Autodesk Inventor part; units mm, degrees
(part 2 of 2)
  line L790 (66.3671, -24) -> (65.1836, -26.05)
  line L791 (65.1836, -26.05) -> (62.8164, -26.05)
  line L792 (62.8164, -26.05) -> (61.6329, -24)
  line L793 (61.6329, -24) -> (62.8164, -21.95)
  circle A263 centre (64, -24) radius 1.1
  circle A264 centre (64, -32) radius 2.05
  line L794 (62.8164, -29.95) -> (65.1836, -29.95)
  line L795 (65.1836, -29.95) -> (66.3671, -32)
  line L796 (66.3671, -32) -> (65.1836, -34.05)
  line L797 (65.1836, -34.05) -> (62.8164, -34.05)
  line L798 (62.8164, -34.05) -> (61.6329, -32)
  line L799 (61.6329, -32) -> (62.8164, -29.95)
  circle A265 centre (64, -32) radius 1.1
  circle A266 centre (64, -40) radius 2.05
  line L800 (62.8164, -37.95) -> (65.1836, -37.95)
  line L801 (65.1836, -37.95) -> (66.3671, -40)
  line L802 (66.3671, -40) -> (65.1836, -42.05)
  line L803 (65.1836, -42.05) -> (62.8164, -42.05)
  line L804 (62.8164, -42.05) -> (61.6329, -40)
  line L805 (61.6329, -40) -> (62.8164, -37.95)
  circle A267 centre (64, -40) radius 1.1
  circle A268 centre (64, -48) radius 2.05
  line L806 (62.8164, -45.95) -> (65.1836, -45.95)
  line L807 (65.1836, -45.95) -> (66.3671, -48)
  line L808 (66.3671, -48) -> (65.1836, -50.05)
  line L809 (65.1836, -50.05) -> (62.8164, -50.05)
  line L810 (62.8164, -50.05) -> (61.6329, -48)
  line L811 (61.6329, -48) -> (62.8164, -45.95)
  circle A269 centre (64, -48) radius 1.1
  circle A270 centre (64, -56) radius 2.05
  line L812 (62.8164, -53.95) -> (65.1836, -53.95)
  line L813 (65.1836, -53.95) -> (66.3671, -56)
  line L814 (66.3671, -56) -> (65.1836, -58.05)
  line L815 (65.1836, -58.05) -> (62.8164, -58.05)
  line L816 (62.8164, -58.05) -> (61.6329, -56)
  line L817 (61.6329, -56) -> (62.8164, -53.95)
  circle A271 centre (64, -56) radius 1.1
  circle A272 centre (64, -64) radius 2.05
  line L818 (62.8164, -61.95) -> (65.1836, -61.95)
  line L819 (65.1836, -61.95) -> (66.3671, -64)
  line L820 (66.3671, -64) -> (65.1836, -66.05)
  line L821 (65.1836, -66.05) -> (62.8164, -66.05)
  line L822 (62.8164, -66.05) -> (61.6329, -64)
  line L823 (61.6329, -64) -> (62.8164, -61.95)
  circle A273 centre (64, -64) radius 1.1
  circle A274 centre (64, -72) radius 2.05
  line L824 (62.8164, -69.95) -> (65.1836, -69.95)
  line L825 (65.1836, -69.95) -> (66.3671, -72)
  line L826 (66.3671, -72) -> (65.1836, -74.05)
  line L827 (65.1836, -74.05) -> (62.8164, -74.05)
  line L828 (62.8164, -74.05) -> (61.6329, -72)
  line L829 (61.6329, -72) -> (62.8164, -69.95)
  circle A275 centre (64, -72) radius 1.1
  circle A276 centre (64, -80) radius 2.05
  line L830 (62.8164, -77.95) -> (65.1836, -77.95)
  line L831 (65.1836, -77.95) -> (66.3671, -80)
  line L832 (66.3671, -80) -> (65.1836, -82.05)
  line L833 (65.1836, -82.05) -> (62.8164, -82.05)
  line L834 (62.8164, -82.05) -> (61.6329, -80)
  line L835 (61.6329, -80) -> (62.8164, -77.95)
  circle A277 centre (64, -80) radius 1.1
  circle A278 centre (64, -88) radius 2.05
  line L836 (62.8164, -85.95) -> (65.1836, -85.95)
  line L837 (65.1836, -85.95) -> (66.3671, -88)
  line L838 (66.3671, -88) -> (65.1836, -90.05)
  line L839 (65.1836, -90.05) -> (62.8164, -90.05)
  line L840 (62.8164, -90.05) -> (61.6329, -88)
  line L841 (61.6329, -88) -> (62.8164, -85.95)
  circle A279 centre (64, -88) radius 1.1
  circle A280 centre (64, -96) radius 2.05
  line L842 (62.8164, -93.95) -> (65.1836, -93.95)
  line L843 (65.1836, -93.95) -> (66.3671, -96)
  line L844 (66.3671, -96) -> (65.1836, -98.05)
  line L845 (65.1836, -98.05) -> (62.8164, -98.05)
  line L846 (62.8164, -98.05) -> (61.6329, -96)
  line L847 (61.6329, -96) -> (62.8164, -93.95)
  circle A281 centre (64, -96) radius 1.1
  circle A282 centre (64, -104) radius 2.05
  line L848 (62.8164, -101.95) -> (65.1836, -101.95)
  line L849 (65.1836, -101.95) -> (66.3671, -104)
  line L850 (66.3671, -104) -> (65.1836, -106.05)
  line L851 (65.1836, -106.05) -> (62.8164, -106.05)
  line L852 (62.8164, -106.05) -> (61.6329, -104)
  line L853 (61.6329, -104) -> (62.8164, -101.95)
  circle A283 centre (64, -104) radius 1.1
  circle A284 centre (64, -112) radius 2.05
  line L854 (62.8164, -109.95) -> (65.1836, -109.95)
  line L855 (65.1836, -109.95) -> (66.3671, -112)
  line L856 (66.3671, -112) -> (65.1836, -114.05)
  line L857 (65.1836, -114.05) -> (62.8164, -114.05)
  line L858 (62.8164, -114.05) -> (61.6329, -112)
  line L859 (61.6329, -112) -> (62.8164, -109.95)
  circle A285 centre (64, -112) radius 1.1
  circle A286 centre (64, -120) radius 2.05
  line L860 (62.8164, -117.95) -> (65.1836, -117.95)
  line L861 (65.1836, -117.95) -> (66.3671, -120)
  line L862 (66.3671, -120) -> (65.1836, -122.05)
  line L863 (65.1836, -122.05) -> (62.8164, -122.05)
  line L864 (62.8164, -122.05) -> (61.6329, -120)
  line L865 (61.6329, -120) -> (62.8164, -117.95)
  circle A287 centre (64, -120) radius 1.1
  circle A288 centre (72, 0) radius 2.05
  line L866 (70.8164, 2.05) -> (73.1836, 2.05)
  line L867 (73.1836, 2.05) -> (74.3671, 0)
  line L868 (74.3671, 0) -> (73.1836, -2.05)
  line L869 (73.1836, -2.05) -> (70.8164, -2.05)
  line L870 (70.8164, -2.05) -> (69.6329, 0)
  line L871 (69.6329, 0) -> (70.8164, 2.05)
  circle A289 centre (72, 0) radius 1.1
  circle A290 centre (72, -8) radius 2.05
  line L872 (70.8164, -5.95) -> (73.1836, -5.95)
  line L873 (73.1836, -5.95) -> (74.3671, -8)
  line L874 (74.3671, -8) -> (73.1836, -10.05)
  line L875 (73.1836, -10.05) -> (70.8164, -10.05)
  line L876 (70.8164, -10.05) -> (69.6329, -8)
  line L877 (69.6329, -8) -> (70.8164, -5.95)
  circle A291 centre (72, -8) radius 1.1
  circle A292 centre (72, -16) radius 2.05
  line L878 (70.8164, -13.95) -> (73.1836, -13.95)
  line L879 (73.1836, -13.95) -> (74.3671, -16)
  line L880 (74.3671, -16) -> (73.1836, -18.05)
  line L881 (73.1836, -18.05) -> (70.8164, -18.05)
  line L882 (70.8164, -18.05) -> (69.6329, -16)
  line L883 (69.6329, -16) -> (70.8164, -13.95)
  circle A293 centre (72, -16) radius 1.1
  circle A294 centre (72, -24) radius 2.05
  line L884 (70.8164, -21.95) -> (73.1836, -21.95)
  line L885 (73.1836, -21.95) -> (74.3671, -24)
  line L886 (74.3671, -24) -> (73.1836, -26.05)
  line L887 (73.1836, -26.05) -> (70.8164, -26.05)
  line L888 (70.8164, -26.05) -> (69.6329, -24)
  line L889 (69.6329, -24) -> (70.8164, -21.95)
  circle A295 centre (72, -24) radius 1.1
  circle A296 centre (72, -32) radius 2.05
  line L890 (70.8164, -29.95) -> (73.1836, -29.95)
  line L891 (73.1836, -29.95) -> (74.3671, -32)
  line L892 (74.3671, -32) -> (73.1836, -34.05)
  line L893 (73.1836, -34.05) -> (70.8164, -34.05)
  line L894 (70.8164, -34.05) -> (69.6329, -32)
  line L895 (69.6329, -32) -> (70.8164, -29.95)
  circle A297 centre (72, -32) radius 1.1
  circle A298 centre (72, -40) radius 2.05
  line L896 (70.8164, -37.95) -> (73.1836, -37.95)
  line L897 (73.1836, -37.95) -> (74.3671, -40)
  line L898 (74.3671, -40) -> (73.1836, -42.05)
  line L899 (73.1836, -42.05) -> (70.8164, -42.05)
  line L900 (70.8164, -42.05) -> (69.6329, -40)
  line L901 (69.6329, -40) -> (70.8164, -37.95)
  circle A299 centre (72, -40) radius 1.1
  circle A300 centre (72, -48) radius 2.05
  line L902 (70.8164, -45.95) -> (73.1836, -45.95)
  line L903 (73.1836, -45.95) -> (74.3671, -48)
  line L904 (74.3671, -48) -> (73.1836, -50.05)
  line L905 (73.1836, -50.05) -> (70.8164, -50.05)
  line L906 (70.8164, -50.05) -> (69.6329, -48)
  line L907 (69.6329, -48) -> (70.8164, -45.95)
  circle A301 centre (72, -48) radius 1.1
  circle A302 centre (72, -56) radius 2.05
  line L908 (70.8164, -53.95) -> (73.1836, -53.95)
  line L909 (73.1836, -53.95) -> (74.3671, -56)
  line L910 (74.3671, -56) -> (73.1836, -58.05)
  line L911 (73.1836, -58.05) -> (70.8164, -58.05)
  line L912 (70.8164, -58.05) -> (69.6329, -56)
  line L913 (69.6329, -56) -> (70.8164, -53.95)
  circle A303 centre (72, -56) radius 1.1
  circle A304 centre (72, -64) radius 2.05
  line L914 (70.8164, -61.95) -> (73.1836, -61.95)
  line L915 (73.1836, -61.95) -> (74.3671, -64)
  line L916 (74.3671, -64) -> (73.1836, -66.05)
  line L917 (73.1836, -66.05) -> (70.8164, -66.05)
  line L918 (70.8164, -66.05) -> (69.6329, -64)
  line L919 (69.6329, -64) -> (70.8164, -61.95)
  circle A305 centre (72, -64) radius 1.1
  circle A306 centre (72, -72) radius 2.05
  line L920 (70.8164, -69.95) -> (73.1836, -69.95)
  line L921 (73.1836, -69.95) -> (74.3671, -72)
  line L922 (74.3671, -72) -> (73.1836, -74.05)
  line L923 (73.1836, -74.05) -> (70.8164, -74.05)
  line L924 (70.8164, -74.05) -> (69.6329, -72)
  line L925 (69.6329, -72) -> (70.8164, -69.95)
  circle A307 centre (72, -72) radius 1.1
  circle A308 centre (72, -80) radius 2.05
  line L926 (70.8164, -77.95) -> (73.1836, -77.95)
  line L927 (73.1836, -77.95) -> (74.3671, -80)
  line L928 (74.3671, -80) -> (73.1836, -82.05)
  line L929 (73.1836, -82.05) -> (70.8164, -82.05)
  line L930 (70.8164, -82.05) -> (69.6329, -80)
  line L931 (69.6329, -80) -> (70.8164, -77.95)
  circle A309 centre (72, -80) radius 1.1
  circle A310 centre (72, -88) radius 2.05
  line L932 (70.8164, -85.95) -> (73.1836, -85.95)
  line L933 (73.1836, -85.95) -> (74.3671, -88)
  line L934 (74.3671, -88) -> (73.1836, -90.05)
  line L935 (73.1836, -90.05) -> (70.8164, -90.05)
  line L936 (70.8164, -90.05) -> (69.6329, -88)
  line L937 (69.6329, -88) -> (70.8164, -85.95)
  circle A311 centre (72, -88) radius 1.1
  circle A312 centre (72, -96) radius 2.05
  line L938 (70.8164, -93.95) -> (73.1836, -93.95)
  line L939 (73.1836, -93.95) -> (74.3671, -96)
  line L940 (74.3671, -96) -> (73.1836, -98.05)
  line L941 (73.1836, -98.05) -> (70.8164, -98.05)
  line L942 (70.8164, -98.05) -> (69.6329, -96)
  line L943 (69.6329, -96) -> (70.8164, -93.95)
  circle A313 centre (72, -96) radius 1.1
  circle A314 centre (72, -104) radius 2.05
  line L944 (70.8164, -101.95) -> (73.1836, -101.95)
  line L945 (73.1836, -101.95) -> (74.3671, -104)
  line L946 (74.3671, -104) -> (73.1836, -106.05)
  line L947 (73.1836, -106.05) -> (70.8164, -106.05)
  line L948 (70.8164, -106.05) -> (69.6329, -104)
  line L949 (69.6329, -104) -> (70.8164, -101.95)
  circle A315 centre (72, -104) radius 1.1
  circle A316 centre (72, -112) radius 2.05
  line L950 (70.8164, -109.95) -> (73.1836, -109.95)
  line L951 (73.1836, -109.95) -> (74.3671, -112)
  line L952 (74.3671, -112) -> (73.1836, -114.05)
  line L953 (73.1836, -114.05) -> (70.8164, -114.05)
  line L954 (70.8164, -114.05) -> (69.6329, -112)
  line L955 (69.6329, -112) -> (70.8164, -109.95)
  circle A317 centre (72, -112) radius 1.1
  circle A318 centre (72, -120) radius 2.05
  line L956 (70.8164, -117.95) -> (73.1836, -117.95)
  line L957 (73.1836, -117.95) -> (74.3671, -120)
  line L958 (74.3671, -120) -> (73.1836, -122.05)
  line L959 (73.1836, -122.05) -> (70.8164, -122.05)
  line L960 (70.8164, -122.05) -> (69.6329, -120)
  line L961 (69.6329, -120) -> (70.8164, -117.95)
  circle A319 centre (72, -120) radius 1.1
  circle A320 centre (80, 0) radius 2.05
  line L962 (78.8164, 2.05) -> (81.1836, 2.05)
  line L963 (81.1836, 2.05) -> (82.3671, 0)
  line L964 (82.3671, 0) -> (81.1836, -2.05)
  line L965 (81.1836, -2.05) -> (78.8164, -2.05)
  line L966 (78.8164, -2.05) -> (77.6329, 0)
  line L967 (77.6329, 0) -> (78.8164, 2.05)
  circle A321 centre (80, 0) radius 1.1
  circle A322 centre (80, -8) radius 2.05
  line L968 (78.8164, -5.95) -> (81.1836, -5.95)
  line L969 (81.1836, -5.95) -> (82.3671, -8)
  line L970 (82.3671, -8) -> (81.1836, -10.05)
  line L971 (81.1836, -10.05) -> (78.8164, -10.05)
  line L972 (78.8164, -10.05) -> (77.6329, -8)
  line L973 (77.6329, -8) -> (78.8164, -5.95)
  circle A323 centre (80, -8) radius 1.1
  circle A324 centre (80, -16) radius 2.05
  line L974 (78.8164, -13.95) -> (81.1836, -13.95)
  line L975 (81.1836, -13.95) -> (82.3671, -16)
  line L976 (82.3671, -16) -> (81.1836, -18.05)
  line L977 (81.1836, -18.05) -> (78.8164, -18.05)
  line L978 (78.8164, -18.05) -> (77.6329, -16)
  line L979 (77.6329, -16) -> (78.8164, -13.95)
  circle A325 centre (80, -16) radius 1.1
  circle A326 centre (80, -24) radius 2.05
  line L980 (78.8164, -21.95) -> (81.1836, -21.95)
  line L981 (81.1836, -21.95) -> (82.3671, -24)
  line L982 (82.3671, -24) -> (81.1836, -26.05)
  line L983 (81.1836, -26.05) -> (78.8164, -26.05)
  line L984 (78.8164, -26.05) -> (77.6329, -24)
  line L985 (77.6329, -24) -> (78.8164, -21.95)
  circle A327 centre (80, -24) radius 1.1
  circle A328 centre (80, -32) radius 2.05
  line L986 (78.8164, -29.95) -> (81.1836, -29.95)
  line L987 (81.1836, -29.95) -> (82.3671, -32)
  line L988 (82.3671, -32) -> (81.1836, -34.05)
  line L989 (81.1836, -34.05) -> (78.8164, -34.05)
  line L990 (78.8164, -34.05) -> (77.6329, -32)
  line L991 (77.6329, -32) -> (78.8164, -29.95)
  circle A329 centre (80, -32) radius 1.1
  circle A330 centre (80, -40) radius 2.05
  line L992 (78.8164, -37.95) -> (81.1836, -37.95)
  line L993 (81.1836, -37.95) -> (82.3671, -40)
  line L994 (82.3671, -40) -> (81.1836, -42.05)
  line L995 (81.1836, -42.05) -> (78.8164, -42.05)
  line L996 (78.8164, -42.05) -> (77.6329, -40)
  line L997 (77.6329, -40) -> (78.8164, -37.95)
  circle A331 centre (80, -40) radius 1.1
  circle A332 centre (80, -48) radius 2.05
  line L998 (78.8164, -45.95) -> (81.1836, -45.95)
  line L999 (81.1836, -45.95) -> (82.3671, -48)
  line L1000 (82.3671, -48) -> (81.1836, -50.05)
  line L1001 (81.1836, -50.05) -> (78.8164, -50.05)
  line L1002 (78.8164, -50.05) -> (77.6329, -48)
  line L1003 (77.6329, -48) -> (78.8164, -45.95)
  circle A333 centre (80, -48) radius 1.1
  circle A334 centre (80, -56) radius 2.05
  line L1004 (78.8164, -53.95) -> (81.1836, -53.95)
  line L1005 (81.1836, -53.95) -> (82.3671, -56)
  line L1006 (82.3671, -56) -> (81.1836, -58.05)
  line L1007 (81.1836, -58.05) -> (78.8164, -58.05)
  line L1008 (78.8164, -58.05) -> (77.6329, -56)
  line L1009 (77.6329, -56) -> (78.8164, -53.95)
  circle A335 centre (80, -56) radius 1.1
  circle A336 centre (80, -64) radius 2.05
  line L1010 (78.8164, -61.95) -> (81.1836, -61.95)
  line L1011 (81.1836, -61.95) -> (82.3671, -64)
  line L1012 (82.3671, -64) -> (81.1836, -66.05)
  line L1013 (81.1836, -66.05) -> (78.8164, -66.05)
  line L1014 (78.8164, -66.05) -> (77.6329, -64)
  line L1015 (77.6329, -64) -> (78.8164, -61.95)
  circle A337 centre (80, -64) radius 1.1
  circle A338 centre (80, -72) radius 2.05
  line L1016 (78.8164, -69.95) -> (81.1836, -69.95)
  line L1017 (81.1836, -69.95) -> (82.3671, -72)
  line L1018 (82.3671, -72) -> (81.1836, -74.05)
  line L1019 (81.1836, -74.05) -> (78.8164, -74.05)
  line L1020 (78.8164, -74.05) -> (77.6329, -72)
  line L1021 (77.6329, -72) -> (78.8164, -69.95)
  circle A339 centre (80, -72) radius 1.1
  circle A340 centre (80, -80) radius 2.05
  line L1022 (78.8164, -77.95) -> (81.1836, -77.95)
  line L1023 (81.1836, -77.95) -> (82.3671, -80)
  line L1024 (82.3671, -80) -> (81.1836, -82.05)
  line L1025 (81.1836, -82.05) -> (78.8164, -82.05)
  line L1026 (78.8164, -82.05) -> (77.6329, -80)
  line L1027 (77.6329, -80) -> (78.8164, -77.95)
  circle A341 centre (80, -80) radius 1.1
  circle A342 centre (80, -88) radius 2.05
  line L1028 (78.8164, -85.95) -> (81.1836, -85.95)
  line L1029 (81.1836, -85.95) -> (82.3671, -88)
  line L1030 (82.3671, -88) -> (81.1836, -90.05)
  line L1031 (81.1836, -90.05) -> (78.8164, -90.05)
  line L1032 (78.8164, -90.05) -> (77.6329, -88)
  line L1033 (77.6329, -88) -> (78.8164, -85.95)
  circle A343 centre (80, -88) radius 1.1
  circle A344 centre (80, -96) radius 2.05
  line L1034 (78.8164, -93.95) -> (81.1836, -93.95)
  line L1035 (81.1836, -93.95) -> (82.3671, -96)
  line L1036 (82.3671, -96) -> (81.1836, -98.05)
  line L1037 (81.1836, -98.05) -> (78.8164, -98.05)
  line L1038 (78.8164, -98.05) -> (77.6329, -96)
  line L1039 (77.6329, -96) -> (78.8164, -93.95)
  circle A345 centre (80, -96) radius 1.1
  circle A346 centre (80, -104) radius 2.05
  line L1040 (78.8164, -101.95) -> (81.1836, -101.95)
  line L1041 (81.1836, -101.95) -> (82.3671, -104)
  line L1042 (82.3671, -104) -> (81.1836, -106.05)
  line L1043 (81.1836, -106.05) -> (78.8164, -106.05)
  line L1044 (78.8164, -106.05) -> (77.6329, -104)
  line L1045 (77.6329, -104) -> (78.8164, -101.95)
  circle A347 centre (80, -104) radius 1.1
  circle A348 centre (80, -112) radius 2.05
  line L1046 (78.8164, -109.95) -> (81.1836, -109.95)
  line L1047 (81.1836, -109.95) -> (82.3671, -112)
  line L1048 (82.3671, -112) -> (81.1836, -114.05)
  line L1049 (81.1836, -114.05) -> (78.8164, -114.05)
  line L1050 (78.8164, -114.05) -> (77.6329, -112)
  line L1051 (77.6329, -112) -> (78.8164, -109.95)
  circle A349 centre (80, -112) radius 1.1
  circle A350 centre (80, -120) radius 2.05
  line L1052 (78.8164, -117.95) -> (81.1836, -117.95)
  line L1053 (81.1836, -117.95) -> (82.3671, -120)
  line L1054 (82.3671, -120) -> (81.1836, -122.05)
  line L1055 (81.1836, -122.05) -> (78.8164, -122.05)
  line L1056 (78.8164, -122.05) -> (77.6329, -120)
  line L1057 (77.6329, -120) -> (78.8164, -117.95)
  circle A351 centre (80, -120) radius 1.1
  circle A352 centre (88, 0) radius 2.05
  line L1058 (86.8164, 2.05) -> (89.1836, 2.05)
  line L1059 (89.1836, 2.05) -> (90.3671, 0)
  line L1060 (90.3671, 0) -> (89.1836, -2.05)
  line L1061 (89.1836, -2.05) -> (86.8164, -2.05)
  line L1062 (86.8164, -2.05) -> (85.6329, 0)
  line L1063 (85.6329, 0) -> (86.8164, 2.05)
  circle A353 centre (88, 0) radius 1.1
  circle A354 centre (88, -8) radius 2.05
  line L1064 (86.8164, -5.95) -> (89.1836, -5.95)
  line L1065 (89.1836, -5.95) -> (90.3671, -8)
  line L1066 (90.3671, -8) -> (89.1836, -10.05)
  line L1067 (89.1836, -10.05) -> (86.8164, -10.05)
  line L1068 (86.8164, -10.05) -> (85.6329, -8)
  line L1069 (85.6329, -8) -> (86.8164, -5.95)
  circle A355 centre (88, -8) radius 1.1
  circle A356 centre (88, -16) radius 2.05
  line L1070 (86.8164, -13.95) -> (89.1836, -13.95)
  line L1071 (89.1836, -13.95) -> (90.3671, -16)
  line L1072 (90.3671, -16) -> (89.1836, -18.05)
  line L1073 (89.1836, -18.05) -> (86.8164, -18.05)
  line L1074 (86.8164, -18.05) -> (85.6329, -16)
  line L1075 (85.6329, -16) -> (86.8164, -13.95)
  circle A357 centre (88, -16) radius 1.1
  circle A358 centre (88, -24) radius 2.05
  line L1076 (86.8164, -21.95) -> (89.1836, -21.95)
  line L1077 (89.1836, -21.95) -> (90.3671, -24)
  line L1078 (90.3671, -24) -> (89.1836, -26.05)
  line L1079 (89.1836, -26.05) -> (86.8164, -26.05)
  line L1080 (86.8164, -26.05) -> (85.6329, -24)
  line L1081 (85.6329, -24) -> (86.8164, -21.95)
  circle A359 centre (88, -24) radius 1.1
  circle A360 centre (88, -32) radius 2.05
  line L1082 (86.8164, -29.95) -> (89.1836, -29.95)
  line L1083 (89.1836, -29.95) -> (90.3671, -32)
  line L1084 (90.3671, -32) -> (89.1836, -34.05)
  line L1085 (89.1836, -34.05) -> (86.8164, -34.05)
  line L1086 (86.8164, -34.05) -> (85.6329, -32)
  line L1087 (85.6329, -32) -> (86.8164, -29.95)
  circle A361 centre (88, -32) radius 1.1
  circle A362 centre (88, -40) radius 2.05
  line L1088 (86.8164, -37.95) -> (89.1836, -37.95)
  line L1089 (89.1836, -37.95) -> (90.3671, -40)
  line L1090 (90.3671, -40) -> (89.1836, -42.05)
  line L1091 (89.1836, -42.05) -> (86.8164, -42.05)
  line L1092 (86.8164, -42.05) -> (85.6329, -40)
  line L1093 (85.6329, -40) -> (86.8164, -37.95)
  circle A363 centre (88, -40) radius 1.1
  circle A364 centre (88, -48) radius 2.05
  line L1094 (86.8164, -45.95) -> (89.1836, -45.95)
  line L1095 (89.1836, -45.95) -> (90.3671, -48)
  line L1096 (90.3671, -48) -> (89.1836, -50.05)
  line L1097 (89.1836, -50.05) -> (86.8164, -50.05)
  line L1098 (86.8164, -50.05) -> (85.6329, -48)
  line L1099 (85.6329, -48) -> (86.8164, -45.95)
  circle A365 centre (88, -48) radius 1.1
  circle A366 centre (88, -56) radius 2.05
  line L1100 (86.8164, -53.95) -> (89.1836, -53.95)
  line L1101 (89.1836, -53.95) -> (90.3671, -56)
  line L1102 (90.3671, -56) -> (89.1836, -58.05)
  line L1103 (89.1836, -58.05) -> (86.8164, -58.05)
  line L1104 (86.8164, -58.05) -> (85.6329, -56)
  line L1105 (85.6329, -56) -> (86.8164, -53.95)
  circle A367 centre (88, -56) radius 1.1
  circle A368 centre (88, -64) radius 2.05
  line L1106 (86.8164, -61.95) -> (89.1836, -61.95)
  line L1107 (89.1836, -61.95) -> (90.3671, -64)
  line L1108 (90.3671, -64) -> (89.1836, -66.05)
  line L1109 (89.1836, -66.05) -> (86.8164, -66.05)
  line L1110 (86.8164, -66.05) -> (85.6329, -64)
  line L1111 (85.6329, -64) -> (86.8164, -61.95)
  circle A369 centre (88, -64) radius 1.1
  circle A370 centre (88, -72) radius 2.05
  line L1112 (86.8164, -69.95) -> (89.1836, -69.95)
  line L1113 (89.1836, -69.95) -> (90.3671, -72)
  line L1114 (90.3671, -72) -> (89.1836, -74.05)
  line L1115 (89.1836, -74.05) -> (86.8164, -74.05)
  line L1116 (86.8164, -74.05) -> (85.6329, -72)
  line L1117 (85.6329, -72) -> (86.8164, -69.95)
  circle A371 centre (88, -72) radius 1.1
  circle A372 centre (88, -80) radius 2.05
  line L1118 (86.8164, -77.95) -> (89.1836, -77.95)
  line L1119 (89.1836, -77.95) -> (90.3671, -80)
  line L1120 (90.3671, -80) -> (89.1836, -82.05)
  line L1121 (89.1836, -82.05) -> (86.8164, -82.05)
  line L1122 (86.8164, -82.05) -> (85.6329, -80)
  line L1123 (85.6329, -80) -> (86.8164, -77.95)
  circle A373 centre (88, -80) radius 1.1
  circle A374 centre (88, -88) radius 2.05
  line L1124 (86.8164, -85.95) -> (89.1836, -85.95)
  line L1125 (89.1836, -85.95) -> (90.3671, -88)
  line L1126 (90.3671, -88) -> (89.1836, -90.05)
  line L1127 (89.1836, -90.05) -> (86.8164, -90.05)
  line L1128 (86.8164, -90.05) -> (85.6329, -88)
  line L1129 (85.6329, -88) -> (86.8164, -85.95)
  circle A375 centre (88, -88) radius 1.1
  circle A376 centre (88, -96) radius 2.05
  line L1130 (86.8164, -93.95) -> (89.1836, -93.95)
  line L1131 (89.1836, -93.95) -> (90.3671, -96)
  line L1132 (90.3671, -96) -> (89.1836, -98.05)
  line L1133 (89.1836, -98.05) -> (86.8164, -98.05)
  line L1134 (86.8164, -98.05) -> (85.6329, -96)
  line L1135 (85.6329, -96) -> (86.8164, -93.95)
  circle A377 centre (88, -96) radius 1.1
  circle A378 centre (88, -104) radius 2.05
  line L1136 (86.8164, -101.95) -> (89.1836, -101.95)
  line L1137 (89.1836, -101.95) -> (90.3671, -104)
  line L1138 (90.3671, -104) -> (89.1836, -106.05)
  line L1139 (89.1836, -106.05) -> (86.8164, -106.05)
  line L1140 (86.8164, -106.05) -> (85.6329, -104)
  line L1141 (85.6329, -104) -> (86.8164, -101.95)
  circle A379 centre (88, -104) radius 1.1
  circle A380 centre (88, -112) radius 2.05
  line L1142 (86.8164, -109.95) -> (89.1836, -109.95)
  line L1143 (89.1836, -109.95) -> (90.3671, -112)
  line L1144 (90.3671, -112) -> (89.1836, -114.05)
  line L1145 (89.1836, -114.05) -> (86.8164, -114.05)
  line L1146 (86.8164, -114.05) -> (85.6329, -112)
  line L1147 (85.6329, -112) -> (86.8164, -109.95)
  circle A381 centre (88, -112) radius 1.1
  circle A382 centre (88, -120) radius 2.05
  line L1148 (86.8164, -117.95) -> (89.1836, -117.95)
  line L1149 (89.1836, -117.95) -> (90.3671, -120)
  line L1150 (90.3671, -120) -> (89.1836, -122.05)
  line L1151 (89.1836, -122.05) -> (86.8164, -122.05)
  line L1152 (86.8164, -122.05) -> (85.6329, -120)
  line L1153 (85.6329, -120) -> (86.8164, -117.95)
  circle A383 centre (88, -120) radius 1.1
  circle A384 centre (96, 0) radius 2.05
  line L1154 (94.8164, 2.05) -> (97.1836, 2.05)
  line L1155 (97.1836, 2.05) -> (98.3671, 0)
  line L1156 (98.3671, 0) -> (97.1836, -2.05)
  line L1157 (97.1836, -2.05) -> (94.8164, -2.05)
  line L1158 (94.8164, -2.05) -> (93.6329, 0)
  line L1159 (93.6329, 0) -> (94.8164, 2.05)
  circle A385 centre (96, 0) radius 1.1
  circle A386 centre (96, -8) radius 2.05
  line L1160 (94.8164, -5.95) -> (97.1836, -5.95)
  line L1161 (97.1836, -5.95) -> (98.3671, -8)
  line L1162 (98.3671, -8) -> (97.1836, -10.05)
  line L1163 (97.1836, -10.05) -> (94.8164, -10.05)
  line L1164 (94.8164, -10.05) -> (93.6329, -8)
  line L1165 (93.6329, -8) -> (94.8164, -5.95)
  circle A387 centre (96, -8) radius 1.1
  circle A388 centre (96, -16) radius 2.05
  line L1166 (94.8164, -13.95) -> (97.1836, -13.95)
  line L1167 (97.1836, -13.95) -> (98.3671, -16)
  line L1168 (98.3671, -16) -> (97.1836, -18.05)
  line L1169 (97.1836, -18.05) -> (94.8164, -18.05)
  line L1170 (94.8164, -18.05) -> (93.6329, -16)
  line L1171 (93.6329, -16) -> (94.8164, -13.95)
  circle A389 centre (96, -16) radius 1.1
  circle A390 centre (96, -24) radius 2.05
  line L1172 (94.8164, -21.95) -> (97.1836, -21.95)
  line L1173 (97.1836, -21.95) -> (98.3671, -24)
  line L1174 (98.3671, -24) -> (97.1836, -26.05)
  line L1175 (97.1836, -26.05) -> (94.8164, -26.05)
  line L1176 (94.8164, -26.05) -> (93.6329, -24)
  line L1177 (93.6329, -24) -> (94.8164, -21.95)
  circle A391 centre (96, -24) radius 1.1
  circle A392 centre (96, -32) radius 2.05
  line L1178 (94.8164, -29.95) -> (97.1836, -29.95)
  line L1179 (97.1836, -29.95) -> (98.3671, -32)
  line L1180 (98.3671, -32) -> (97.1836, -34.05)
  line L1181 (97.1836, -34.05) -> (94.8164, -34.05)
  line L1182 (94.8164, -34.05) -> (93.6329, -32)
  line L1183 (93.6329, -32) -> (94.8164, -29.95)
  circle A393 centre (96, -32) radius 1.1
  circle A394 centre (96, -40) radius 2.05
  line L1184 (94.8164, -37.95) -> (97.1836, -37.95)
  line L1185 (97.1836, -37.95) -> (98.3671, -40)
  line L1186 (98.3671, -40) -> (97.1836, -42.05)
  line L1187 (97.1836, -42.05) -> (94.8164, -42.05)
  line L1188 (94.8164, -42.05) -> (93.6329, -40)
  line L1189 (93.6329, -40) -> (94.8164, -37.95)
  circle A395 centre (96, -40) radius 1.1
  circle A396 centre (96, -48) radius 2.05
  line L1190 (94.8164, -45.95) -> (97.1836, -45.95)
  line L1191 (97.1836, -45.95) -> (98.3671, -48)
  line L1192 (98.3671, -48) -> (97.1836, -50.05)
  line L1193 (97.1836, -50.05) -> (94.8164, -50.05)
  line L1194 (94.8164, -50.05) -> (93.6329, -48)
  line L1195 (93.6329, -48) -> (94.8164, -45.95)
  circle A397 centre (96, -48) radius 1.1
  circle A398 centre (96, -56) radius 2.05
  line L1196 (94.8164, -53.95) -> (97.1836, -53.95)
  line L1197 (97.1836, -53.95) -> (98.3671, -56)
  line L1198 (98.3671, -56) -> (97.1836, -58.05)
  line L1199 (97.1836, -58.05) -> (94.8164, -58.05)
  line L1200 (94.8164, -58.05) -> (93.6329, -56)
  line L1201 (93.6329, -56) -> (94.8164, -53.95)
  circle A399 centre (96, -56) radius 1.1
  circle A400 centre (96, -64) radius 2.05
  line L1202 (94.8164, -61.95) -> (97.1836, -61.95)
  line L1203 (97.1836, -61.95) -> (98.3671, -64)
  line L1204 (98.3671, -64) -> (97.1836, -66.05)
  line L1205 (97.1836, -66.05) -> (94.8164, -66.05)
  line L1206 (94.8164, -66.05) -> (93.6329, -64)
  line L1207 (93.6329, -64) -> (94.8164, -61.95)
  circle A401 centre (96, -64) radius 1.1
  circle A402 centre (96, -72) radius 2.05
  line L1208 (94.8164, -69.95) -> (97.1836, -69.95)
  line L1209 (97.1836, -69.95) -> (98.3671, -72)
  line L1210 (98.3671, -72) -> (97.1836, -74.05)
  line L1211 (97.1836, -74.05) -> (94.8164, -74.05)
  line L1212 (94.8164, -74.05) -> (93.6329, -72)
  line L1213 (93.6329, -72) -> (94.8164, -69.95)
  circle A403 centre (96, -72) radius 1.1
  circle A404 centre (96, -80) radius 2.05
  line L1214 (94.8164, -77.95) -> (97.1836, -77.95)
  line L1215 (97.1836, -77.95) -> (98.3671, -80)
  line L1216 (98.3671, -80) -> (97.1836, -82.05)
  line L1217 (97.1836, -82.05) -> (94.8164, -82.05)
  line L1218 (94.8164, -82.05) -> (93.6329, -80)
  line L1219 (93.6329, -80) -> (94.8164, -77.95)
  circle A405 centre (96, -80) radius 1.1
  circle A406 centre (96, -88) radius 2.05
  line L1220 (94.8164, -85.95) -> (97.1836, -85.95)
  line L1221 (97.1836, -85.95) -> (98.3671, -88)
  line L1222 (98.3671, -88) -> (97.1836, -90.05)
  line L1223 (97.1836, -90.05) -> (94.8164, -90.05)
  line L1224 (94.8164, -90.05) -> (93.6329, -88)
  line L1225 (93.6329, -88) -> (94.8164, -85.95)
  circle A407 centre (96, -88) radius 1.1
  circle A408 centre (96, -96) radius 2.05
  line L1226 (94.8164, -93.95) -> (97.1836, -93.95)
  line L1227 (97.1836, -93.95) -> (98.3671, -96)
  line L1228 (98.3671, -96) -> (97.1836, -98.05)
  line L1229 (97.1836, -98.05) -> (94.8164, -98.05)
  line L1230 (94.8164, -98.05) -> (93.6329, -96)
  line L1231 (93.6329, -96) -> (94.8164, -93.95)
  circle A409 centre (96, -96) radius 1.1
  circle A410 centre (96, -104) radius 2.05
  line L1232 (94.8164, -101.95) -> (97.1836, -101.95)
  line L1233 (97.1836, -101.95) -> (98.3671, -104)
  line L1234 (98.3671, -104) -> (97.1836, -106.05)
  line L1235 (97.1836, -106.05) -> (94.8164, -106.05)
  line L1236 (94.8164, -106.05) -> (93.6329, -104)
  line L1237 (93.6329, -104) -> (94.8164, -101.95)
  circle A411 centre (96, -104) radius 1.1
  circle A412 centre (96, -112) radius 2.05
  line L1238 (94.8164, -109.95) -> (97.1836, -109.95)
  line L1239 (97.1836, -109.95) -> (98.3671, -112)
  line L1240 (98.3671, -112) -> (97.1836, -114.05)
  line L1241 (97.1836, -114.05) -> (94.8164, -114.05)
  line L1242 (94.8164, -114.05) -> (93.6329, -112)
  line L1243 (93.6329, -112) -> (94.8164, -109.95)
  circle A413 centre (96, -112) radius 1.1
  circle A414 centre (96, -120) radius 2.05
  line L1244 (94.8164, -117.95) -> (97.1836, -117.95)
  line L1245 (97.1836, -117.95) -> (98.3671, -120)
  line L1246 (98.3671, -120) -> (97.1836, -122.05)
  line L1247 (97.1836, -122.05) -> (94.8164, -122.05)
  line L1248 (94.8164, -122.05) -> (93.6329, -120)
  line L1249 (93.6329, -120) -> (94.8164, -117.95)
  circle A415 centre (96, -120) radius 1.1
  dimension "d8" = 4.1
  dimension "d16" = 2.2
  dimension "d17" = 3
  dimension "d20" = 8
  dimension "d23" = 8
  constraints: 2500 end point, 416 centre point, 208 coincident, 6 tangent, 3 parallel, 2 equal length, 2 horizontal, 2 vertical, 1 perpendicular, 3312 other
  measures "d8" diameter of A0
  measures "d16" diameter of A1
  measures "d17" distance of L6.start L6.end
  measures "d20" distance of A0.centre A2.centre
  measures "d23" distance of A0.centre A32.centre
sketch "스케치2" plane through (0, 0, 0) normal (0, 1, 0) x (-1, 0, 0)
  line L0 (-4, 4) -> (100, 4)
  line L1 (100, 4) -> (100, -124)
  line L2 (100, -124) -> (-4, -124)
  line L3 (-4, -124) -> (-4, 4)
  point P0 (0, 0)
  dimension "d28" = 104
  dimension "d29" = 128
  constraints: 8 end point, 2 parallel, 1 horizontal, 1 perpendicular
  measures "d28" distance of L1.end L2.end
  measures "d29" distance of L0.end L1.end
extrude "돌출1" add sketch "스케치2" against normal blind 5
fillet "모깎기1" radius 3 4 edges at (-100, -2.5, -124) (-100, -2.5, 4) (4, -2.5, -124) (4, -2.5, 4)
extrude "돌출2" cut sketch "스케치1" against normal blind 5 contours A1
extrude "돌출3" cut sketch "스케치1" against normal blind 3 contours A0 | A0 L1 L2 | A0 L0 L1 | L2 L3 A0 | A0 L5 L0 | L3 L4 A0 | A0 L4 L5 | A1
pattern_linear "직사각형 패턴1" count 16 spacing 8 along (0, 0, -1) count 13 spacing 8 along (-1, 0, 0) of "돌출3", "돌출2"
equation "\"TransitionRadius\" = BendRadius"
equation "\"BendRadius\" = 0.5"
